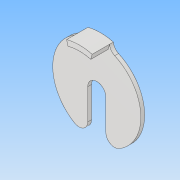
# Autodesk Inventor part: SpoolSpacer
Saved by Autodesk Inventor 2017.3 (Build 213256000, 256)
## iProperties
Created: 2019-06-29
Part Number: SpoolSpacer
Material: ABS Plastic
Document SubType Name: Modeling
Designer: Derek Wider
Density: 1.06 g/cm^3
Appearance: Smooth - White
Author: Derek Wider
Autodesk Inventor part; units mm, degrees
ref_plane "YZ Plane" through (0, 0, 0) normal (1, 0, 0) x (0, 1, 0)
ref_plane "XZ Plane" through (0, 0, 0) normal (0, 1, 0) x (-1, 0, 0)
ref_plane "XY Plane" through (0, 0, 0) normal (0, 0, 1) x (1, 0, 0)
sketch "Sketch1" plane through (0, 0, 0) normal (0, 0, 1) x (1, 0, 0)
  arc A0 (3.302, 0) -> (-3.302, 0) centre (0, 0) ccw
  arc A1 (3.302, -15.7225) -> (-3.302, -15.7225) centre (0, 0) ccw
  line L0 (-3.302, 0) -> (-3.302, -15.7225)
  line L1 (3.302, 0) -> (3.302, -15.7225)
  dimension "d0" = 6.604
  dimension "d1" = 32.131
  constraints: 4 end point, 4 point on circle, 2 centre point, 2 tangent, 2 vertical, 1 coincident, 1 concentric
  measures "d0" diameter of A0
  measures "d1" diameter of A1
extrude "Extrusion1" add sketch "Sketch1" along normal blind 1.397
sketch "Sketch2" plane through (0, 0, 1.397) normal (0, 0, 1) x (1, 0, 0)
  arc A0 (3.302, 0) -> (-3.302, 0) centre (0, 0) ccw projected
  line L0 (3.302, 0) -> (3.302, -15.7225) projected
  arc A1 (3.302, -15.7225) -> (-3.302, -15.7225) centre (0, 0) ccw projected
  line L1 (-3.302, -15.7225) -> (-3.302, 0) projected
  arc A2 (3.302, -15.7225) -> (-3.302, -15.7225) centre (0, 0) ccw projected
  line L2 (-4.1581, 15.5181) -> (-4.6511, 17.3582)
  line L3 (4.1581, 15.5181) -> (4.6511, 17.3582)
  arc A3 (4.6511, 17.3582) -> (-4.6511, 17.3582) centre (0, 0) ccw
  line L4 (-4.1581, 15.5181) -> (4.1581, 15.5181) construction
  dimension "d6" = 1.905
  dimension "d7" = 30
  constraints: 6 end point, 6 point on circle, 2 line through centre, 1 centre point, 1 coincident, 1 equal length, 1 horizontal
  measures "d6" distance of L2.start L2.end
extrude "Extrusion2" add sketch "Sketch2" along normal blind 6.35 and the other way blind 1.397 contours A1 L2 A3 L3
fillet "Fillet1" radius 3.175 4 edges at (4.1581, 15.5181, 0.6985) (-4.1581, 15.5181, 0.6985) (-3.302, -15.7225, 0.6985) (3.302, -15.7225, 0.6985)
body "Solid1"
